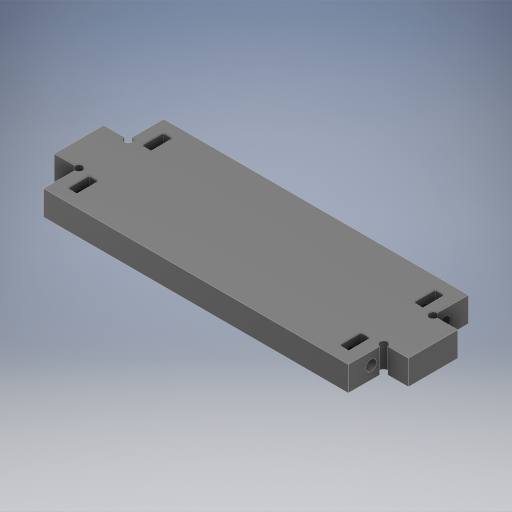
# Autodesk Inventor part: chest connection
Saved by Autodesk Inventor 2024 (Build 280153000, 153)
## iProperties
Created: 2024-09-05
Part Number: chest connection
Material: PMMA 플라스틱
Document SubType Name: Modeling
Designer: msi
Density: 1.188 g/cm^3
Appearance: 매끄러움 - 검은색
Author: msi
Autodesk Inventor part; units mm, degrees
ref_plane "우측면도" through (0, 0, 0) normal (1, 0, 0) x (0, 1, 0)
ref_plane "평면도" through (0, 0, 0) normal (0, 1, 0) x (-1, 0, 0)
ref_plane "정면도" through (0, 0, 0) normal (0, 0, 1) x (1, 0, 0)
sketch "스케치1" plane through (0, 0, 0) normal (0, 1, 0) x (-1, 0, 0)
  line L0 (-37, 14.6) -> (37, 14.6)
  line L1 (37, 14.6) -> (37, -14.6)
  line L2 (37, -14.6) -> (-37, -14.6)
  line L3 (-37, -14.6) -> (-37, 14.6)
  line L4 (-37, 14.6) -> (37, -14.6) construction
  line L5 (37, 14.6) -> (-37, -14.6) construction
  line L6 (37, 6) -> (43, 6)
  line L7 (43, 6) -> (43, -6)
  line L8 (43, -6) -> (37, -6)
  line L9 (37, -6) -> (37, 6)
  line L10 (-37, 6) -> (-43, 6)
  line L11 (-43, 6) -> (-43, -6)
  line L12 (-43, -6) -> (-37, -6)
  line L13 (-37, -6) -> (-37, 6)
  point P0 (0, 0)
  dimension "d0" = 74
  dimension "d1" = 29.2
  dimension "d2" = 6
  dimension "d3" = 12
  dimension "d4" = 6
  dimension "d5" = 12
  constraints: 28 end point, 6 parallel, 3 horizontal, 3 perpendicular, 2 midpoint, 2 point on line
  measures "d0" distance of L1.end L2.end
  measures "d1" distance of L0.end L1.end
  measures "d2" distance of L7.end L8.end
  measures "d3" distance of L6.end L7.end
  measures "d4" distance of L12.end L11.end
  measures "d5" distance of L11.end L10.end
extrude "돌출1" add sketch "스케치1" along normal blind 6
sketch "스케치2" plane through (43, 0, 6) normal (1, 0, 0) x (0, 0, -1)
  line L0 (12, 0) -> (20.6, 0) projected
  line L1 (20.6, 0) -> (20.6, 6) projected
  line L2 (12, 6) -> (20.6, 6) projected
  line L3 (12, 0) -> (12, 6) projected
  line L4 (-8.6, 0) -> (0, 0) projected
  line L5 (0, 0) -> (0, 6) projected
  line L6 (-8.6, 6) -> (0, 6) projected
  line L7 (-8.6, 0) -> (-8.6, 6) projected
  circle A0 centre (15, 3) radius 1.35
  circle A1 centre (-3, 3) radius 1.35
  point P0 (6, 0)
  dimension "d8" = 2.7
  dimension "d9" = 2.7
  constraints: 2 centre point
  measures "d8" diameter of A0
  measures "d9" diameter of A1
extrude "돌출2" cut sketch "스케치2" against normal blind 14 contours A0 | A1
sketch "스케치3" plane through (-43, 0, -6) normal (-1, 0, 0) x (0, 0, 1)
  line L0 (12, 0) -> (20.6, 0) projected
  line L1 (20.6, 0) -> (20.6, 6) projected
  line L2 (12, 6) -> (20.6, 6) projected
  line L3 (12, 0) -> (12, 6) projected
  circle A0 centre (-3, 3) radius 1.35 projected
  line L4 (-8.6, 0) -> (0, 0) projected
  line L5 (0, 0) -> (0, 6) projected
  line L6 (-8.6, 6) -> (0, 6) projected
  line L7 (-8.6, 0) -> (-8.6, 6) projected
  circle A1 centre (15, 3) radius 1.35 projected
  circle A2 centre (-3, 3) radius 1.35
  circle A3 centre (15, 3) radius 1.35
  point P0 (6, 0)
  constraints: 2 centre point, 2 coincident, 2 concentric
extrude "돌출3" cut sketch "스케치3" against normal blind 14 contours A0 | A1
sketch "스케치4" plane through (0, 6, 0) normal (0, 1, 0) x (1, 0, 0)
  line L0 (37, -14.6) -> (37, -6) projected
  line L1 (37, -6) -> (43, -6) projected
  line L2 (43, -6) -> (43, 6) projected
  line L3 (43, 6) -> (37, 6) projected
  line L4 (37, 6) -> (37, 14.6) projected
  line L5 (37, 14.6) -> (-37, 14.6) projected
  line L6 (-37, 14.6) -> (-37, 6) projected
  line L7 (-37, 6) -> (-43, 6) projected
  line L8 (-43, 6) -> (-43, -6) projected
  line L9 (-43, -6) -> (-37, -6) projected
  line L10 (-37, -6) -> (-37, -14.6) projected
  line L11 (-37, -14.6) -> (37, -14.6) projected
  line L12 (-37, 10.35) -> (-29, 10.35) projected
  line L13 (-37, 7.65) -> (-29, 7.65) projected
  line L14 (-33, 10.35) -> (-33, 7.65)
  line L15 (-34.1, 6.4) -> (-31.9, 6.4)
  line L16 (-31.9, 6.4) -> (-31.9, 11.6)
  line L17 (-31.9, 11.6) -> (-34.1, 11.6)
  line L18 (-34.1, 11.6) -> (-34.1, 6.4)
  line L19 (-34.1, 6.4) -> (-31.9, 11.6) construction
  line L20 (-31.9, 6.4) -> (-34.1, 11.6) construction
  line L21 (34.1, 6.4) -> (31.9, 6.4)
  line L22 (31.9, 6.4) -> (31.9, 11.6)
  line L23 (31.9, 11.6) -> (34.1, 11.6)
  line L24 (34.1, 11.6) -> (34.1, 6.4)
  line L25 (34.1, 6.4) -> (31.9, 11.6) construction
  line L26 (31.9, 6.4) -> (34.1, 11.6) construction
  line L27 (31.9, -11.6) -> (34.1, -11.6)
  line L28 (34.1, -11.6) -> (34.1, -6.4)
  line L29 (34.1, -6.4) -> (31.9, -6.4)
  line L30 (31.9, -6.4) -> (31.9, -11.6)
  line L31 (31.9, -11.6) -> (34.1, -6.4) construction
  line L32 (34.1, -11.6) -> (31.9, -6.4) construction
  line L33 (-34.1, -11.6) -> (-31.9, -11.6)
  line L34 (-31.9, -11.6) -> (-31.9, -6.4)
  line L35 (-31.9, -6.4) -> (-34.1, -6.4)
  line L36 (-34.1, -6.4) -> (-34.1, -11.6)
  line L37 (-34.1, -11.6) -> (-31.9, -6.4) construction
  line L38 (-31.9, -11.6) -> (-34.1, -6.4) construction
  point P0 (0, 0)
  point P1 (-33, 9)
  point P2 (33, 9)
  point P3 (33, -9)
  point P4 (-33, -9)
  dimension "d14" = 2.2
  dimension "d15" = 5.2
  dimension "d16" = 2.2
  dimension "d17" = 5.2
  dimension "d18" = 2.2
  dimension "d19" = 5.2
  dimension "d20" = 2.2
  dimension "d21" = 5.2
  constraints: 50 end point, 11 midpoint, 8 parallel, 4 horizontal, 4 perpendicular
  measures "d14" distance of L17.end L16.end
  measures "d15" distance of L16.end L15.end
  measures "d16" distance of L22.end L23.end
  measures "d17" distance of L21.end L22.end
  measures "d18" distance of L29.end L28.end
  measures "d19" distance of L28.end L27.end
  measures "d20" distance of L35.end L34.end
  measures "d21" distance of L34.end L33.end
extrude "돌출4" cut sketch "스케치4" against normal blind 14 contours L18 L12 L14 L13 | L13 L16 L15 L18 | L18 L17 L16 L12 | L14 L12 L16 L13 | L21 L22 L23 L24 | L30 L29 L28 L27 | L36 L35 L34 L33
sketch "스케치5" plane through (0, 6, 0) normal (0, 1, 0) x (1, 0, 0)
  line L0 (31.9, 6.4) -> (31.9, 11.6) projected
  line L1 (31.9, 11.6) -> (34.1, 11.6) projected
  line L2 (34.1, 11.6) -> (34.1, 6.4) projected
  line L3 (34.1, 6.4) -> (31.9, 6.4) projected
  line L4 (-34.1, -6.4) -> (-31.9, -6.4) projected
  line L5 (-31.9, -6.4) -> (-31.9, -11.6) projected
  line L6 (-31.9, -11.6) -> (-34.1, -11.6) projected
  line L7 (-34.1, -11.6) -> (-34.1, -6.4) projected
  line L8 (31.9, -6.4) -> (34.1, -6.4) projected
  line L9 (34.1, -6.4) -> (34.1, -11.6) projected
  line L10 (34.1, -11.6) -> (31.9, -11.6) projected
  line L11 (31.9, -11.6) -> (31.9, -6.4) projected
  line L12 (-34.1, 6.4) -> (-34.1, 11.6) projected
  line L13 (-34.1, 11.6) -> (-31.9, 11.6) projected
  line L14 (-31.9, 11.6) -> (-31.9, 6.4) projected
  line L15 (-31.9, 6.4) -> (-34.1, 6.4) projected
  line L16 (37, -14.6) -> (37, -6) projected
  line L17 (37, -6) -> (43, -6) projected
  line L18 (43, -6) -> (43, 6) projected
  line L19 (43, 6) -> (37, 6) projected
  line L20 (37, 6) -> (37, 14.6) projected
  line L21 (37, 14.6) -> (-37, 14.6) projected
  line L22 (-37, 14.6) -> (-37, 6) projected
  line L23 (-37, 6) -> (-43, 6) projected
  line L24 (-43, 6) -> (-43, -6) projected
  line L25 (-43, -6) -> (-37, -6) projected
  line L26 (-37, -6) -> (-37, -14.6) projected
  line L27 (-37, -14.6) -> (37, -14.6) projected
  circle A0 centre (-37, -6) radius 1
  circle A1 centre (-37, 6) radius 1
  circle A2 centre (37, -6) radius 1
  circle A3 centre (37, 6) radius 1
  point P0 (0, 0)
  point P1 (-37, -7)
  point P2 (-38, -6)
  dimension "d24" = 2
  dimension "d25" = 2
  dimension "d26" = 2
  dimension "d27" = 2
  constraints: 4 centre point, 4 coincident
  measures "d24" diameter of A0
  measures "d25" diameter of A1
  measures "d26" diameter of A2
  measures "d27" diameter of A3
extrude "돌출5" cut sketch "스케치5" against normal through all contours A2 L17 L16 | L16 L17 A2 | L26 L25 A0 | A3 L20 L19 | L19 L20 A3 | A1 L22 L23 | L23 L22 A1 picked at (-37.657, -5.9202)
